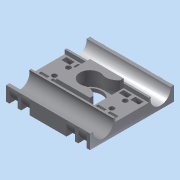
# Autodesk Inventor part: Extruder Mount
Saved by Autodesk Inventor 2015 (Build 190159000, 159)
## iProperties
Created: 2016-06-25
Part Number: Extruder Mount
Material: Generic
Document SubType Name: Modeling
Designer: Dustin
Density: 1 g/cm^3
Appearance: Default
Mass: 14.8984 g
Surface Area: 87.5211 cm^2
Volume: 14.8984 cm^3
Author: Dustin
Autodesk Inventor part; units mm, degrees
ref_plane "YZ Plane" through (0, 0, 0) normal (1, 0, 0) x (0, 1, 0)
ref_plane "XZ Plane" through (0, 0, 0) normal (0, 1, 0) x (-1, 0, 0)
ref_plane "XY Plane" through (0, 0, 0) normal (0, 0, 1) x (1, 0, 0)
sketch "Sketch1" plane through (0, 0, 0) normal (0, 1, 0) x (-1, 0, 0)
  point P0 (0, 0)
sketch "Sketch2" plane through (0, 0, 0) normal (0, 1, 0) x (-1, 0, 0)
  line L0 (0, 0) -> (20, 0)
  line L1 (20, 0) -> (20, -20)
  line L2 (20, -20) -> (0, -20)
  line L3 (0, -20) -> (0, 0)
  point P0 (10, -10)
  dimension "d0" = 20
  dimension "d1" = 20
  dimension "d2" = 10
  dimension "d12" = 10
  constraints: 8 end point, 2 parallel, 1 horizontal, 1 perpendicular
  measures "d0" distance of L2.end L0.start
  measures "d1" distance of L0.start L0.end
  measures "d2" distance from line of L1 point (10, -10)
  measures "d12" distance from line of L2 point (10, -10)
extrude "Extrusion1" add sketch "Sketch2" along normal blind 6
sketch "Sketch3" plane through (0, 0, 0) normal (0, -1, 0) x (1, 0, 0)
  point P0 (0, 0)
  point P1 (-10, -10)
hole "Hole1" at (-10, 0, -10) direction (0, 1, 0) diameter 12 depth 25.4 tip angle 118
sketch "Sketch4" plane through (0, 0, 0) normal (0, -1, 0) x (1, 0, 0)
  circle A0 centre (-10, -10) radius 6 projected
  line L0 (0, 0) -> (0, -20) projected
  arc A1 (-7.3025, -4.6405) -> (0, -2) centre (-5.8808, 2.8456) ccw
  arc A2 (0, -18) -> (-7.2265, -15.3205) centre (-5.8987, -22.8239) ccw
  arc A3 (-7.2265, -15.3205) -> (-7.3025, -4.6405) centre (-10, -10) ccw
  line L1 (0, -2) -> (0, -18)
  dimension "d13" = 2
  dimension "d14" = 2
  dimension "d16" = 7.62
  dimension "d17" = 7.62
  constraints: 8 point on circle, 3 centre point, 2 end point, 2 point on line, 1 collinear, 1 concentric
  measures "d13" distance of L0.start L1.start
  measures "d14" distance of L0.end L1.end
  measures "d16" radius of A1
  measures "d17" radius of A2
extrude "Extrusion2" cut sketch "Sketch4" against normal blind 6 contours A0 A1 L0 A2
sketch "Sketch5" plane through (0, 0, 0) normal (0, -1, 0) x (1, 0, 0)
  circle A0 centre (-10, -10) radius 8
  line L0 (0, 0) -> (-20, 0)
  line L1 (-20, 0) -> (-20, -20)
  line L2 (-20, -20) -> (0, -20)
  line L3 (-10, -2) -> (0, -2)
  line L4 (-10, -18) -> (0, -18)
  line L5 (0, 0) -> (0, -2)
  line L6 (0, -2) -> (0, 0) projected
  line L7 (0, -18) -> (0, -20)
  dimension "d20" = 16
  constraints: 14 end point, 3 horizontal, 2 equal length, 2 point on circle, 1 centre point, 1 coincident, 1 perpendicular, 1 tangent, 1 vertical
  measures "d20" diameter of A0
extrude "Extrusion3" add sketch "Sketch5" along normal blind 4 contours A0 L4 L7 L2 L1 L0 L5 L3
sketch "Sketch6" plane through (0, -4, 0) normal (0, -1, 0) x (1, 0, 0)
  line L0 (-35, -35) -> (15, -35)
  line L1 (15, -35) -> (15, 15)
  line L2 (15, 15) -> (-35, 15)
  line L3 (-35, 15) -> (-35, -35)
  line L4 (-20, 0) -> (-20, -20) projected
  line L5 (-20, -20) -> (0, -20) projected
  point P0 (0, 0)
  point P1 (-10, -10)
  dimension "d32" = 50
  dimension "d33" = 50
  dimension "d34" = 15
  dimension "d35" = 15
  constraints: 8 end point, 2 parallel, 1 horizontal, 1 perpendicular
  measures "d32" distance of L2.end L0.start
  measures "d33" distance of L0.start L0.end
  measures "d34" distance between parallel lines of L4 L3
  measures "d35" distance between parallel lines of L0 L5
extrude "Extrusion4" add sketch "Sketch6" along normal blind 4
sketch "Sketch7" plane through (0, -4, 0) normal (0, 1, 0) x (1, 0, 0)
  point P0 (0, 0)
  point P1 (-10, 10)
hole "Hole2" at (-10, -4, -10) direction (0, -1, 0) diameter 14 depth 25.4 tip angle 118
sketch "Sketch8" plane through (-35, -4, -35) normal (-1, 0, 0) x (0, 0, 1)
  circle A0 centre (42, 6) radius 6
  line L0 (50, 0) -> (50, -4) projected
  circle A1 centre (8, 6) radius 6
  line L1 (50, 0) -> (0, 0) projected
  line L2 (0, 0) -> (0, -4) projected
  line L3 (15, 0) -> (0, 0)
  line L4 (0, 0) -> (0, 6.51)
  line L5 (0, 6.51) -> (2.0217, 6.51)
  line L6 (13.8258, 7.4353) -> (15, 7.4353)
  line L7 (15, 10) -> (15, 0) projected
  line L8 (15, 7.4353) -> (15, 0)
  arc A2 (2.0217, 6.51) -> (2.0217, 6.51) centre (7.9748, 6.0021) ccw
  line L9 (47.9783, 6.51) -> (50, 6.51)
  line L10 (50, 6.51) -> (50, 0)
  line L11 (50, 0) -> (35, 0)
  line L12 (0, 0) -> (50, 0) projected
  line L13 (35, 10) -> (35, 0) projected
  line L14 (35, 7.4593) -> (36.1802, 7.4593)
  arc A3 (36.1802, 7.4593) -> (47.9783, 6.51) centre (42, 6) ccw
  point P0 (35, 4)
  dimension "d36" = 12
  dimension "d37" = 8
  dimension "d38" = 12
  dimension "d39" = 6
  dimension "d40" = 6
  dimension "d41" = 8
  constraints: 18 end point, 10 point on circle, 4 centre point, 4 perpendicular, 3 horizontal, 3 point on line, 2 tangent, 1 collinear, 1 concentric
  measures "d36" diameter of A0
  measures "d37" distance from line of L0 A0.centre
  measures "d38" diameter of A1
  measures "d39" distance from line of L1 A0.centre
  measures "d40" distance from line of L1 A1.centre
  measures "d41" distance from line of L2 A1.centre
extrude "Extrusion5" add sketch "Sketch8" against normal up to surface (50 mm away) contours A0 L9 L10 L1 | L1 L13 L14 A0 | A1 L6 L7 L1 | L1 L4 L5 A1
sketch "Sketch9" plane through (0, -8, 0) normal (0, -1, 0) x (1, 0, 0)
  line L0 (15, -35) -> (15, 15) projected
  line L1 (0, 0) -> (15, 0) projected
  line L2 (15, -20) -> (0, -20) projected
  line L3 (-35, 15) -> (-35, -35) projected
  line L4 (-35, 0) -> (-20, 0) projected
  line L5 (-35, -21.1742) -> (15, -21.1742) projected
  line L6 (-35, 1.1802) -> (15, 1.1802) projected
  point P0 (7, -6)
  point P1 (7, -14)
  point P2 (-27, -5.8198)
  point P3 (-27, -14.1742)
  dimension "d44" = 8
  dimension "d45" = 8
  dimension "d46" = 6
  dimension "d47" = 6
  dimension "d55" = 8
  dimension "d56" = 8
  dimension "d79" = 7
  dimension "d94" = 7
  measures "d44" distance from line of L0 point (7, -6)
  measures "d45" distance from line of L0 point (7, -14)
  measures "d46" distance from line of L1 point (7, -6)
  measures "d47" distance from line of L2 point (7, -14)
  measures "d55" distance from line of L3 point (-27, -5.82)
  measures "d56" distance from line of L3 point (-27, -14.174)
  measures "d79" distance from line of L5 point (-27, -14.174)
  measures "d94" distance from line of point (-27, -5.82) L6
hole "Hole3" at (7, -8, -14) at (7, -8, -6) at (-27, -8, -5.8198) at (-27, -8, -14.1742) direction (0, 1, 0) diameter 3 depth 25.4 tip angle 118
sketch "Sketch10" plane through (-35, -8, -35) normal (-1, 0, 0) x (0, 0, 1)
  line L0 (0, 10.51) -> (0, 0) projected
  line L1 (50, 0) -> (0, 0)
  line L2 (0, 0) -> (0, 2)
  line L3 (0, 2) -> (50, 2)
  line L4 (50, 2) -> (50, 0)
  point P0 (35, 8)
  dimension "d57" = 2
  constraints: 8 end point, 2 parallel, 1 horizontal, 1 perpendicular, 1 point on line
  measures "d57" distance of L3.end L1.start
extrude "Extrusion6" cut sketch "Sketch10" against normal through all
sketch "Sketch11" plane through (0, -4, 0) normal (0, 1, 0) x (1, 0, 0)
  circle A0 centre (-27, 5.8198) radius 1.5 projected
  circle A1 centre (-27, 14.1742) radius 1.5 projected
  line L0 (-20, 20) -> (-35, 20) projected
  line L1 (-35, 0) -> (-35, 20) projected
  line L2 (-35, 0) -> (-20, 0) projected
  line L3 (-20, 0) -> (-20, 20) projected
  circle A2 centre (7, 14) radius 1.5 projected
  circle A3 centre (7, 6) radius 1.5 projected
  circle A4 centre (-10, 10) radius 7 projected
  line L4 (15, 20) -> (0, 20) projected
  line L5 (0, 20) -> (0, 18) projected
  line L6 (0, 18) -> (-10, 18) projected
  arc A5 (-10, 18) -> (-10, 2) centre (-10, 10) ccw projected
  line L7 (-10, 2) -> (0, 2) projected
  line L8 (0, 2) -> (0, 0) projected
  line L9 (0, 0) -> (15, 0) projected
  line L10 (15, 20) -> (15, 0) projected
  line L11 (15, 0) -> (0, 0)
  line L12 (0, 0) -> (0, 20)
  line L13 (0, 20) -> (15, 20)
  line L14 (15, 20) -> (15, 0)
  point P0 (0, 0)
  constraints: 8 end point, 2 parallel, 1 horizontal, 1 perpendicular
extrude "Extrusion7" add sketch "Sketch11" along normal blind 5 contours L3 L2 L1 L0 | L10 L9 L8 L12 L5 L4
sketch "Sketch12" plane through (15, 2.51, -32.9783) normal (1, 0, 0) x (0, 0, -1)
  arc A0 (-45.9566, 0) -> (-34.1585, 0.9493) centre (-39.9783, -0.51) ccw projected
  circle A1 centre (-39.9783, -0.51) radius 8.5
  circle A2 centre (-39.9783, -0.51) radius 10.5
  point P0 (-32.9783, -2.51)
  dimension "d62" = 17
  dimension "d63" = 2
  constraints: 2 centre point, 2 coincident
  measures "d62" diameter of A1
  measures "d63" radial gap between concentric circles of A2 A1
extrude "Extrusion9" add sketch "Sketch12" against normal blind 1
sketch "Sketch13" plane through (15, 2.51, -32.9783) normal (1, 0, 0) x (0, 0, -1)
  line L0 (-31.5373, -1.51) -> (-29.526, -1.51)
  line L1 (-31.5373, -1.51) -> (-29.526, -1.51) projected
  line L2 (-37.106, -8.51) -> (-33.1776, -8.51)
  line L3 (-33.1776, -8.51) -> (-37.106, -8.51) projected
  line L4 (-47.9783, -8.51) -> (-33.1776, -8.51)
  line L5 (2.0217, -8.51) -> (-47.9783, -8.51) projected
  line L6 (-47.9783, -8.51) -> (-47.9783, 0)
  line L7 (-47.9783, -8.51) -> (-31.832, -8.51)
  line L8 (-31.832, -8.51) -> (-31.832, -14.5869)
  line L9 (-31.832, -14.5869) -> (-47.9783, -14.5869)
  line L10 (-47.9783, -14.5869) -> (-47.9783, -8.51)
  line L11 (-47.9783, -8.51) -> (-51.7546, -8.51)
  line L12 (-51.7546, -8.51) -> (-51.7546, 6.9564)
  line L13 (-51.7546, 6.9564) -> (-47.9783, 6.9564)
  line L14 (-47.9783, 6.9564) -> (-47.9783, -8.51)
  line L15 (-47.9783, 0) -> (-27.1599, 0)
  line L16 (-27.1599, 0) -> (-27.1599, 11.1031)
  line L17 (-27.1599, 11.1031) -> (-47.9783, 11.1031)
  line L18 (-47.9783, 11.1031) -> (-47.9783, 0)
  line L19 (-32.9783, -1.51) -> (-27.1599, -1.51)
  line L20 (-27.1599, -1.51) -> (-27.1599, 0)
  line L21 (-27.1599, 0) -> (-32.9783, 0)
  line L22 (-32.9783, 0) -> (-32.9783, -1.51)
  point P0 (-32.9783, -2.51)
  constraints: 40 end point, 8 parallel, 4 horizontal, 4 perpendicular, 3 collinear, 1 vertical
extrude "Extrusion10" cut sketch "Sketch13" against normal blind 1
sketch "Sketch14" plane through (14, 2.51, -32.9783) normal (1, 0, 0) x (0, 0, -1)
  arc A0 (-34, 0) -> (-34.1585, 0.9493) centre (-39.9783, -0.51) ccw projected
  line L0 (-32.9783, 0) -> (-34, 0) projected
  line L1 (-32.9783, 0.9493) -> (-32.9783, 0) projected
  line L2 (-34.1585, 0.9493) -> (-32.9783, 0.9493) projected
  point P0 (-32.9783, -2.51)
extrude "Extrusion11" add sketch "Sketch14" along normal blind 1
sketch "Sketch15" plane through (0, 1, 0) normal (0, 1, 0) x (1, 0, 0)
  line L0 (15, 0) -> (15, 20) projected
  line L1 (15, 1) -> (13, 1)
  line L2 (13, 1) -> (13, 3.4515)
  line L3 (13, 3.4515) -> (15, 3.4515)
  line L4 (15, 3.4515) -> (15, 1)
  line L5 (13, 1) -> (8, 1)
  line L6 (8, 1) -> (8, 4)
  line L7 (8, 4) -> (13, 4)
  line L8 (13, 4) -> (13, 1)
  line L9 (15, -13) -> (15, -1) projected
  line L10 (15, -7) -> (0, -7)
  line L11 (0, 0) -> (15, 0) projected
  point P0 (15, -12.9783)
  point P1 (15, -1.1802)
  dimension "d80" = 2
  dimension "d81" = 5
  dimension "d89" = 3
  dimension "d90" = 1
  constraints: 18 end point, 4 parallel, 3 horizontal, 2 perpendicular, 1 midpoint, 1 point on line
  measures "d80" distance between parallel lines of L0 L2
  measures "d81" distance of L6.end L7.end
  measures "d89" distance of L5.end L6.end
  measures "d90" distance between parallel lines of L5 L11
revolve "Revolution1" cut sketch "Sketch15" angle 360 about axis through (15, 1, 7) along (-1, 0, 0) contours L5 L6 L7 L8 L2
pattern_linear "Rectangular Pattern2" count 2 spacing 7 along (-1, 0, 0) count 2 spacing 34 along (0, 0, -1) of "Revolution1"
pattern_linear "Rectangular Pattern3" count 2 spacing 34 along (-1, 0, 0) of "Revolution1", "Rectangular Pattern2"
body "Solid1"
